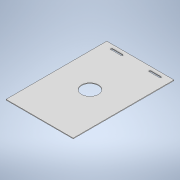
# Autodesk Inventor part: FixedLid
Saved by Autodesk Inventor 2020 (Build 240168000, 168)
## iProperties
Created: 2021-11-12
Part Number: FixedLid
Material: Generic
Document SubType Name: Sheet Metal
Designer: 17185
Density: 1 g/cm^3
Sheet Metal Rule: Default
Appearance: Default
Author: 17185
Autodesk Inventor part; units mm, degrees
ref_plane "YZ Plane" through (0, 0, 0) normal (1, 0, 0) x (0, 1, 0)
ref_plane "XZ Plane" through (0, 0, 0) normal (0, 1, 0) x (-1, 0, 0)
ref_plane "XY Plane" through (0, 0, 0) normal (0, 0, 1) x (1, 0, 0)
sketch "Sketch3" plane through (0, 0, 0) normal (0, 1, 0) x (-1, 0, 0)
  line L0 (152.4, 228.6) -> (-152.4, 228.6)
  line L1 (-152.4, 228.6) -> (-152.4, -228.6)
  line L2 (-152.4, -228.6) -> (152.4, -228.6)
  line L3 (152.4, -228.6) -> (152.4, 228.6)
  line L4 (152.4, 228.6) -> (-152.4, -228.6) construction
  line L5 (-152.4, 228.6) -> (152.4, -228.6) construction
  circle A0 centre (0, 0) radius 38.1
  dimension "d4" = 304.8
  dimension "d5" = 457.2
  dimension "d6" = 76.2
  measures "d4" distance of L1.end L2.end
  measures "d5" distance of L0.end L1.end
  measures "d6" diameter of A0
extrude "Plate2" add sketch "Sketch3" along normal blind 3.048
sketch "Sketch4" plane through (0, 3.048, 0) normal (0, 1, 0) x (1, 0, 0)
  line L0 (-110.49, 208.28) -> (-63.5, 208.28) construction
  line L1 (-110.49, 204.47) -> (-63.5, 204.47)
  line L2 (-63.5, 212.09) -> (-110.49, 212.09)
  arc A0 (-110.49, 212.09) -> (-110.49, 204.47) centre (-110.49, 208.28) ccw
  arc A1 (-63.5, 204.47) -> (-63.5, 212.09) centre (-63.5, 208.28) ccw
  line L3 (152.4, 228.6) -> (-152.4, 228.6) construction
  line L4 (0, 228.6) -> (0, 141.7531) construction
  line L5 (-152.4, -228.6) -> (-152.4, 228.6) projected
  line L6 (110.49, 208.28) -> (63.5, 208.28) construction
  line L7 (110.49, 204.47) -> (63.5, 204.47)
  line L8 (63.5, 212.09) -> (110.49, 212.09)
  arc A2 (110.49, 204.47) -> (110.49, 212.09) centre (110.49, 208.28) ccw
  arc A3 (63.5, 212.09) -> (63.5, 204.47) centre (63.5, 208.28) ccw
  point P0 (0, 0)
  point P1 (-86.995, 208.28)
  point P2 (86.995, 208.28)
  dimension "d8" = 46.99
  dimension "d9" = 7.62
  dimension "d10" = 20.32
  dimension "d11" = 41.91
  constraints: 18 end point, 8 point on circle, 7 symmetric about line, 4 centre point, 4 tangent, 2 midpoint, 1 horizontal, 1 parallel, 1 vertical, 2 other
  measures "d8" distance of L0.start L0.end
  measures "d9" diameter of A1
  measures "d10" distance from line of point (-86.995, 208.28) L3
  measures "d11" distance from line of L0.start L5
extrude "Cut1" cut sketch "Sketch4" against normal blind 3.048
equation "\"d12\" = Thickness"
equation "\"d7\" = Thickness"
equation "\"BendRadius\" = Thickness"
equation "\"BendReliefWidth\" = Thickness"
equation "\"BendReliefDepth\" = 0.5 * Thickness"
equation "\"CornerReliefSize\" = 4 * Thickness"
equation "\"MinimumRemnant\" = 2 * Thickness"
equation "\"TransitionRadius\" = BendRadius"
equation "\"JacobiRadiusSize\" = BendRadius"
equation "\"GapSize\" = Thickness"
equation "\"Thickness\" = 3.048"
body "Solid2"
